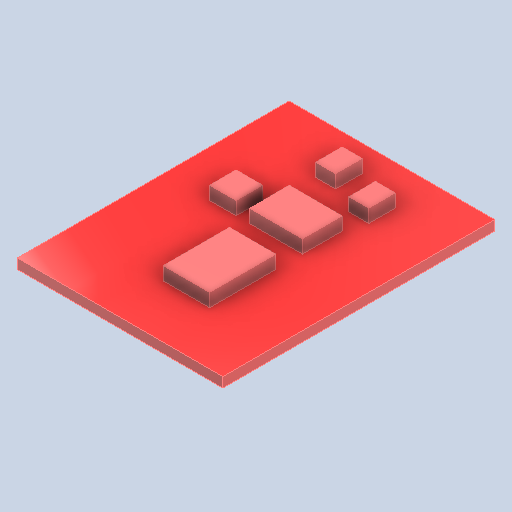
# Autodesk Inventor part: РБАСУ
Saved by Autodesk Inventor 2022 (Build 260153000, 153)
## iProperties
Created: 2022-05-03
Part Number: РБАСУ
Material: Пластик АБС
Document SubType Name: Modeling
Designer: Кочетов.А.И.
Density: 1.06 g/cm^3
Appearance: Гладкий — красный
Author: Кочетов.А.И.
Autodesk Inventor part; units mm, degrees
ref_plane "YZ Plane" through (0, 0, 0) normal (1, 0, 0) x (0, 1, 0)
ref_plane "XZ Plane" through (0, 0, 0) normal (0, 1, 0) x (-1, 0, 0)
ref_plane "XY Plane" through (0, 0, 0) normal (0, 0, 1) x (1, 0, 0)
sketch "Эскиз1" plane through (0, 0, 0) normal (0, 1, 0) x (-1, 0, 0)
  line L0 (-15.5, 20.5) -> (15.5, 20.5)
  line L1 (15.5, 20.5) -> (15.5, -20.5)
  line L2 (15.5, -20.5) -> (-15.5, -20.5)
  line L3 (-15.5, -20.5) -> (-15.5, 20.5)
  line L4 (-15.5, 20.5) -> (15.5, -20.5) construction
  line L5 (15.5, 20.5) -> (-15.5, -20.5) construction
  point P0 (0, 0)
  dimension "d0" = 41
  dimension "d1" = 31
  constraints: 12 end point, 2 midpoint, 2 parallel, 1 horizontal, 1 perpendicular
  measures "d0" distance of L0.end L1.end
  measures "d1" distance of L0.start L0.end
extrude "Выдавливание1" add sketch "Эскиз1" along normal blind 1.5
sketch "Эскиз2" plane through (0, 1.5, 0) normal (0, 1, 0) x (1, 0, 0)
  line L0 (-1.5, -12.5) -> (5.5, -12.5)
  line L1 (5.5, -12.5) -> (5.5, -2.5)
  line L2 (5.5, -2.5) -> (-1.5, -2.5)
  line L3 (-1.5, -2.5) -> (-1.5, -12.5)
  line L4 (-1.5, -12.5) -> (5.5, -2.5) construction
  line L5 (5.5, -12.5) -> (-1.5, -2.5) construction
  line L6 (-2.5, 1.5) -> (5.5, 1.5)
  line L7 (5.5, 1.5) -> (5.5, 7.5)
  line L8 (5.5, 7.5) -> (-2.5, 7.5)
  line L9 (-2.5, 7.5) -> (-2.5, 1.5)
  line L10 (-2.5, 1.5) -> (5.5, 7.5) construction
  line L11 (5.5, 1.5) -> (-2.5, 7.5) construction
  line L12 (3.5, 10.5) -> (6.5, 10.5)
  line L13 (6.5, 10.5) -> (6.5, 14.5)
  line L14 (6.5, 14.5) -> (3.5, 14.5)
  line L15 (3.5, 14.5) -> (3.5, 10.5)
  line L16 (3.5, 10.5) -> (6.5, 14.5) construction
  line L17 (6.5, 10.5) -> (3.5, 14.5) construction
  line L18 (-3.5, 16.5) -> (-0.5, 16.5)
  line L19 (-0.5, 16.5) -> (-0.5, 12.5)
  line L20 (-0.5, 12.5) -> (-3.5, 12.5)
  line L21 (-3.5, 12.5) -> (-3.5, 16.5)
  line L22 (-3.5, 16.5) -> (-0.5, 12.5) construction
  line L23 (-0.5, 16.5) -> (-3.5, 12.5) construction
  line L24 (-8.5, 5.5) -> (-4.5, 5.5)
  line L25 (-4.5, 5.5) -> (-4.5, 1.5)
  line L26 (-4.5, 1.5) -> (-8.5, 1.5)
  line L27 (-8.5, 1.5) -> (-8.5, 5.5)
  line L28 (-8.5, 5.5) -> (-4.5, 1.5) construction
  line L29 (-4.5, 5.5) -> (-8.5, 1.5) construction
  line L30 (15.5, 20.5) -> (-15.5, 20.5) projected
  line L31 (15.5, -20.5) -> (15.5, 20.5) projected
  line L32 (-15.5, -20.5) -> (15.5, -20.5) projected
  point P0 (0, 0)
  point P1 (2, -7.5)
  point P2 (1.5, 4.5)
  point P3 (5, 12.5)
  point P4 (-2, 14.5)
  point P5 (-6.5, 3.5)
  dimension "d4" = 4
  dimension "d5" = 4
  dimension "d6" = 3
  dimension "d7" = 4
  dimension "d8" = 3
  dimension "d9" = 6
  dimension "d10" = 8
  dimension "d11" = 7
  dimension "d12" = 10
  dimension "d13" = 6
  dimension "d14" = 4
  dimension "d15" = 16
  dimension "d16" = 9
  dimension "d17" = 15
  dimension "d18" = 20
  dimension "d19" = 13
  dimension "d20" = 10
  dimension "d21" = 10
  dimension "d22" = 8
  constraints: 60 end point, 10 midpoint, 10 parallel, 6 perpendicular, 5 horizontal
  measures "d4" distance of L26.end L24.start
  measures "d5" distance of L20.end L18.start
  measures "d6" distance of L19.end L20.end
  measures "d7" distance of L14.end L12.start
  measures "d8" distance of L13.end L14.end
  measures "d9" distance of L8.end L6.start
  measures "d10" distance of L7.end L8.end
  measures "d11" distance of L0.start L0.end
  measures "d12" distance of L2.end L0.start
  measures "d13" distance between parallel lines of L30 L14
  measures "d14" distance between parallel lines of L30 L18
  measures "d15" distance between parallel lines of L31 L19
  measures "d16" distance between parallel lines of L31 L13
  measures "d17" distance between parallel lines of L30 L24
  measures "d18" distance between parallel lines of L31 L25
  measures "d19" distance between parallel lines of L30 L8
  measures "d20" distance between parallel lines of L31 L7
  measures "d21" distance between parallel lines of L31 L1
  measures "d22" distance between parallel lines of L32 L0
extrude "Выдавливание2" add sketch "Эскиз2" along normal blind 2
sketch "Эскиз3" plane through (0, 0, 0) normal (0, -1, 0) x (1, 0, 0)
  line L0 (-6.5, -9) -> (9.5, -9)
  line L1 (9.5, -9) -> (9.5, 9)
  line L2 (9.5, 9) -> (-6.5, 9)
  line L3 (-6.5, 9) -> (-6.5, -9)
  line L4 (-6.5, -9) -> (9.5, 9) construction
  line L5 (9.5, -9) -> (-6.5, 9) construction
  line L6 (15.5, 20.5) -> (15.5, -20.5) projected
  line L7 (-10.5, -4) -> (-6.5, -4)
  line L8 (-6.5, -4) -> (-6.5, 4)
  line L9 (-6.5, 4) -> (-10.5, 4)
  line L10 (-10.5, 4) -> (-10.5, -4)
  line L11 (-10.5, -4) -> (-6.5, 4) construction
  line L12 (-6.5, -4) -> (-10.5, 4) construction
  line L13 (-15.5, -20.5) -> (-15.5, 20.5) projected
  point P0 (0, 0)
  point P1 (1.5, 0)
  point P2 (1.5, 0)
  point P3 (-8.5, 0)
  point P4 (-8.5, 0)
  dimension "d25" = 16
  dimension "d26" = 18
  dimension "d27" = 6
  dimension "d28" = 8
  dimension "d29" = 4
  dimension "d30" = 5
  constraints: 24 end point, 6 midpoint, 4 parallel, 2 horizontal, 2 horizontal alignment, 2 perpendicular
  measures "d25" distance of L1.end L2.end
  measures "d26" distance of L2.end L0.start
  measures "d27" distance between parallel lines of L6 L1
  measures "d28" distance of L9.end L7.start
  measures "d29" distance of L8.end L9.end
  measures "d30" distance between parallel lines of L13 L10
extrude "Выдавливание3" add sketch "Эскиз3" along normal blind 5 contours L3 L2 L1 L0
sketch "Эскиз4" plane through (0, 0, 0) normal (0, -1, 0) x (1, 0, 0)
  line L0 (-6.5, 4) -> (-10.5, 4)
  line L1 (-10.5, 4) -> (-10.5, -4)
  line L2 (-10.5, -4) -> (-6.5, -4)
  line L3 (-6.5, -4) -> (-6.5, 4)
  line L4 (-6.5, 4) -> (-10.5, -4) construction
  line L5 (-10.5, 4) -> (-6.5, -4) construction
  line L6 (-15.5, -20.5) -> (-15.5, 20.5) projected
  point P0 (0, 0)
  point P1 (-8.5, 0)
  point P2 (-8.5, 0)
  dimension "d33" = 4
  dimension "d34" = 8
  dimension "d35" = 5
  constraints: 12 end point, 3 midpoint, 2 parallel, 1 horizontal, 1 horizontal alignment, 1 perpendicular
  measures "d33" distance of L1.end L2.end
  measures "d34" distance of L0.end L1.end
  measures "d35" distance between parallel lines of L6 L1
extrude "Выдавливание4" add sketch "Эскиз4" along normal blind 2
